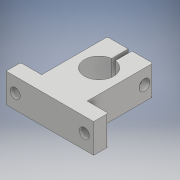
# Autodesk Inventor part: Sk16
Saved by Autodesk Inventor 2018 (Build 220112000, 112)
## iProperties
Created: 2018-09-20
Part Number: Sk16
Material: Genérico
Document SubType Name: Modeling
Designer: Georgines
Density: 1 g/cm^3
Appearance: Padrão
Author: Georgines
Autodesk Inventor part; units mm, degrees
ref_plane "YZ Plane" through (0, 0, 0) normal (1, 0, 0) x (0, 1, 0)
ref_plane "XZ Plane" through (0, 0, 0) normal (0, 1, 0) x (-1, 0, 0)
ref_plane "XY Plane" through (0, 0, 0) normal (0, 0, 1) x (1, 0, 0)
sketch "Esboço1" plane through (0, 0, 0) normal (0, 0, 1) x (1, 0, 0)
  line L0 (23.7277, -0.0451) -> (-24.2723, -0.0451)
  line L1 (-24.2723, -0.0451) -> (-24.2723, 7.9549)
  line L2 (23.7277, 7.9549) -> (23.7277, -0.0451)
  line L3 (12.2277, 43.9549) -> (12.2277, 7.9549)
  line L4 (-12.7723, 7.9549) -> (-12.7723, 43.9549)
  arc A0 (-1.2723, 34.8922) -> (0.7277, 34.8922) centre (-0.2723, 26.9549) ccw
  line L5 (-24.2723, 7.9549) -> (-12.7723, 7.9549)
  line L6 (12.2277, 7.9549) -> (23.7277, 7.9549)
  line L7 (0.7277, 43.9549) -> (0.7277, 34.8922)
  line L8 (-1.2723, 34.8922) -> (-1.2723, 43.9549)
  line L9 (-12.7723, 43.9549) -> (-1.2723, 43.9549)
  line L10 (0.7277, 43.9549) -> (12.2277, 43.9549)
  point P0 (-0.2723, 43.9549)
  dimension "largura" = 48
  dimension "largura_topo" = 25
  dimension "altura_base" = 8
  dimension "diametro" = 16
  dimension "altura_furo" = 27
  dimension "d6" = 11.5
  dimension "d7" = 12.5
  dimension "d8" = 8
  dimension "d10" = 11.5
  dimension "d11" = 11.5
  constraints: 22 end point, 5 parallel, 4 perpendicular, 3 horizontal, 2 point on circle, 1 centre point
  measures "largura" distance of L0.start L0.end
  measures "largura_topo" distance of L4.end L3.start
  measures "altura_base" distance of L0.end L1.end
  measures "diametro" diameter of A0
  measures "altura_furo" distance from line of A0.centre L0
  measures "d6" distance of L1.end L4.start
  measures "d7" distance from line of L4 A0.centre
  measures "d8" distance of L2.start L0.start
  measures "d10" distance of L7.start L3.start
  measures "d11" distance of L4.end L8.end
extrude "Extrusão1" add sketch "Esboço1" along normal blind 16
sketch "Esboço2" plane through (12.2277, 7.9549, 0) normal (1, 0, 0) x (0, 0, -1)
  line L0 (0, 26.9373) -> (-16, 26.9373) projected
  line L1 (-8, 26.9373) -> (-8, 35.7534) construction
  circle A0 centre (-8, 31.3453) radius 1.1711 construction
  point P0 (0, -7.9549)
  constraints: 2 end point, 2 midpoint, 1 centre point, 1 vertical
hole "Furo1" at (12.2277, 39.3003, 8) direction (-1, 0, 0) diameter 3.242 end through all counterbore diameter 6 counterbore depth 4 thread size "M4x0.7" class "6H" standard "ANSI Metric M Profile"
sketch "Esboço3" plane through (-24.2723, -0.0451, 0) normal (0, -1, 0) x (1, 0, 0)
  line L0 (5, 8) -> (43, 8) construction
  circle A0 centre (5, 8) radius 1 construction
  circle A1 centre (43, 8) radius 1 construction
  line L1 (48, 0) -> (0, 0) construction
  line L2 (24, 0) -> (24, 16) construction
  line L3 (0, 16) -> (48, 16) construction
  point P0 (24, 8)
  dimension "distancia_parafusos" = 38
  dimension "d22" = 2
  dimension "d23" = 2
  constraints: 4 end point, 4 midpoint, 2 centre point, 2 coincident, 1 horizontal
  measures "distancia_parafusos" distance of L0.start L0.end
  measures "d22" diameter of A0
  measures "d23" diameter of A1
hole "Furo2" at (-19.2723, -0.0451, 8) at (18.7277, -0.0451, 8) direction (0, 1, 0) diameter 5.5 end through all
fillet "Arredondamento1" radius 1 4 edges at (12.2277, 43.9549, 8) (-12.7723, 43.9549, 8) (-24.2723, 7.9549, 8) (23.7277, 7.9549, 8)
equation "\"d6\" = -0.5 * largura_topo + 0.5 * largura"
equation "\"d7\" = 0.5 * largura_topo"
equation "\"d8\" = altura_base"
equation "\"d11\" = d10"
